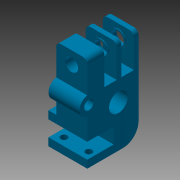
# Autodesk Inventor part: Part3
Saved by Autodesk Inventor 2015 (Build 190159000, 159)
## iProperties
Created: 2015-07-07
Part Number: Part3
Material: ABS Plastic
Document SubType Name: Modeling
Designer: eefred
Density: 1.06 g/cm^3
Appearance: Sky Blue Medium
Author: eefred
Autodesk Inventor part; units mm, degrees
ref_plane "YZ Plane" through (0, 0, 0) normal (1, 0, 0) x (0, 1, 0)
ref_plane "XZ Plane" through (0, 0, 0) normal (0, 1, 0) x (-1, 0, 0)
ref_plane "XY Plane" through (0, 0, 0) normal (0, 0, 1) x (1, 0, 0)
sketch "Sketch1" plane through (0, 0, 0) normal (1, 0, 0) x (0, 1, 0)
  line L0 (0, 0) -> (0, -5)
  line L1 (0, -5) -> (17, -5)
  line L2 (17, -5) -> (17, -15)
  line L3 (17, -15) -> (0, -15)
  line L4 (0, -61) -> (33, -61)
  line L5 (33, -61) -> (33, 0)
  line L6 (33, 0) -> (0, 0)
  circle A0 centre (1, -35) radius 3
  arc A1 (0, -29.0839) -> (0, -40.9161) centre (1, -35) ccw
  line L7 (0, -15) -> (0, -29.0839)
  line L8 (0, -61) -> (0, -40.9161)
  dimension "d0" = 5
  dimension "d1" = 17
  dimension "d2" = 10
  dimension "d4" = 33
  dimension "d6" = 6
  dimension "d7" = 1
  dimension "d8" = 20
  dimension "d9" = 6
  dimension "d49" = 46
  constraints: 18 end point, 5 perpendicular, 3 vertical, 2 centre point, 2 point on circle, 2 point on line, 1 coincident, 1 horizontal
  measures "d0" distance of L0.start L0.end
  measures "d1" distance of L0.end L1.end
  measures "d2" distance of L1.end L2.end
  measures "d4" distance of L4.start L4.end
  measures "d6" diameter of A0
  measures "d7" horizontal distance of L0.start A0.centre
  measures "d8" distance from line of L3 A0.centre
  measures "d9" radius of A1
  measures "d49" distance between parallel lines of L4 L3
extrude "Extrusion1" add sketch "Sketch1" along normal blind 25
sketch "Sketch2" plane through (0, 0, 0) normal (-1, 0, 0) x (0, 0, 1)
  line L0 (-70, -8) -> (-20, -8)
  line L1 (-20, -8) -> (-20, 42)
  line L2 (-20, 42) -> (-70, 42)
  line L3 (-70, 42) -> (-70, -8)
  point P0 (0, 0)
  dimension "d12" = 20
  dimension "d13" = 8
  dimension "d14" = 50
  dimension "d15" = 50
  constraints: 8 end point, 2 parallel, 1 horizontal, 1 perpendicular
  measures "d12" distance from line of point (0, 0) L1
  measures "d13" distance from line of point (0, 0) L0
  measures "d14" distance of L0.start L0.end
  measures "d15" distance of L2.end L0.start
extrude "Extrusion2" cut sketch "Sketch2" against normal blind 5
sketch "Sketch3" plane through (5, 0, 0) normal (-1, 0, 0) x (0, 0, 1)
  line L0 (-61, 22) -> (-40, 22)
  line L1 (-40, 22) -> (-40, 30)
  line L2 (-40, 30) -> (-61, 30)
  line L3 (-61, 30) -> (-61, 22)
  line L4 (-61, 11) -> (-40, 11)
  line L5 (-40, 11) -> (-40, 19)
  line L6 (-40, 19) -> (-61, 19)
  line L7 (-61, 19) -> (-61, 11)
  line L8 (-61, 33) -> (-20, 33) projected
  point P0 (0, 0)
  dimension "d18" = 8
  dimension "d19" = 8
  dimension "d20" = 21
  dimension "d21" = 3
  dimension "d22" = 3
  constraints: 16 end point, 4 parallel, 2 horizontal, 2 perpendicular, 2 point on line, 1 vertical alignment
  measures "d18" distance of L6.end L4.start
  measures "d19" distance of L2.end L0.start
  measures "d20" distance of L1.end L2.end
  measures "d21" distance between parallel lines of L0 L6
  measures "d22" distance between parallel lines of L8 L2
extrude "Extrusion3" cut sketch "Sketch3" against normal up to next
sketch "Sketch4" plane through (0, 33, 0) normal (0, 1, 0) x (1, 0, 0)
  circle A0 centre (15, 53) radius 4.1
  line L0 (5, 61) -> (25, 61) projected
  point P0 (0, 0)
  point P1 (15, 61)
  dimension "d25" = 8.2
  dimension "d26" = 8
  constraints: 1 centre point, 1 midpoint, 1 vertical alignment
  measures "d25" diameter of A0
  measures "d26" distance from line of L0 A0.centre
extrude "Extrusion4" cut sketch "Sketch4" against normal through all
sketch "Sketch5" plane through (5, 11, -40) normal (0, 1, 0) x (1, 0, 0)
  circle A0 centre (10, 13) radius 4.1 projected
  circle A1 centre (10, 13) radius 5
  point P0 (-5, -40)
  dimension "d29" = 10
  constraints: 1 centre point, 1 coincident
  measures "d29" diameter of A1
extrude "Extrusion5" add sketch "Sketch5" along normal blind 0.5
pattern_linear "Rectangular Pattern1" count 2 spacing 11 along (0, 1, 0) of "Extrusion5"
pattern_linear "Rectangular Pattern2" count 2 spacing 7.5 along (0, 1, 0) of "Extrusion5", "Rectangular Pattern1"
sketch "Sketch6" plane through (25, 0, 0) normal (1, 0, 0) x (0, 0, -1)
  circle A0 centre (27, 20) radius 6
  line L0 (61, 33) -> (0, 33) projected
  line L1 (0, 33) -> (0, 0) projected
  dimension "d38" = 12
  dimension "d39" = 13
  dimension "d40" = 27
  constraints: 1 centre point
  measures "d38" diameter of A0
  measures "d39" distance from line of L0 A0.centre
  measures "d40" distance from line of L1 A0.centre
extrude "Extrusion6" cut sketch "Sketch6" against normal up to surface (20 mm away)
fillet "Fillet1" radius 3 6 edges at (25, 31.5, -61) (25, 20.5, -61) (25, 5.5, -61) (5, 31.5, -61) (5, 20.5, -61) (5, 5.5, -61)
fillet "Fillet2" radius 10 1 edges at (12.5, 33, 0)
mirror "Mirror1" about plane through (0, 0, 0) normal (0, 0, 1) remove original yes
sketch "Sketch8" plane through (0, 33, 20) normal (0, 1, 0) x (1, 0, 0)
  line L0 (9.0185, 0.8332) -> (8.8914, 0.7605)
  spline S0 degree 2 poles (8.8914, 0.7605) (8.6371, 0.5971) (8.51, 0.5971) knots 0 0 0 1 1 1
  spline S1 degree 2 poles (8.51, 0.5971) (8.2557, 0.5971) (7.8925, 1.1056) (7.8925, 1.3144) knots 0 0 0 1 2 2 2
  spline S2 degree 2 poles (7.8925, 1.3144) (7.8925, 1.4052) (7.9016, 1.5505) knots 0 0 0 1 1 1
  spline S3 degree 2 poles (7.9016, 1.5505) (7.9288, 1.6958) (7.9288, 1.7321) knots 0 0 0 1 1 1
  spline S4 degree 2 poles (7.9288, 1.7321) (7.6837, 3.2668) (7.6837, 3.8842) knots 0 0 0 1 1 1
  spline S5 degree 2 poles (7.6837, 3.8842) (7.6837, 5.0465) (8.7824, 6.3996) (9.5906, 6.3996) knots 0 0 0 1 2 2 2
  spline S6 degree 2 poles (9.5906, 6.3996) (10.3624, 6.3996) (11.7518, 5.0738) (12.1967, 3.9569) knots 0 0 0 1 2 2 2
  spline S7 degree 2 poles (12.1967, 3.9569) (13.695, 5.8093) (14.258, 6.7719) knots 0 0 0 1 1 1
  spline S8 degree 2 poles (14.258, 6.7719) (14.4578, 7.1078) (14.7756, 7.1078) knots 0 0 0 1 1 1
  spline S9 degree 2 poles (14.7756, 7.1078) (14.9845, 7.1078) (15.4022, 6.6357) (15.4022, 6.4268) knots 0 0 0 1 2 2 2
  spline S10 degree 2 poles (15.4022, 6.4268) (15.4022, 6.1181) (14.8846, 5.3553) (13.7586, 3.9478) (13.6496, 3.8388) knots 0 0 0 1 2 3 3 3
  spline S11 degree 2 poles (13.6496, 3.8388) (12.8233, 2.849) (12.5509, 2.4041) knots 0 0 0 1 1 1
  spline S12 degree 2 poles (12.5509, 2.4041) (12.5509, 1.8593) (12.006, 1.8593) knots 0 0 0 1 1 1
  spline S13 degree 2 poles (12.006, 1.8593) (11.7518, 1.8593) (11.3795, 2.3405) (11.3795, 2.6584) knots 0 0 0 1 2 2 2
  spline S14 degree 2 poles (11.3795, 2.6584) (11.3795, 2.7492) (11.4067, 2.849) knots 0 0 0 1 1 1
  spline S15 degree 2 poles (11.4067, 2.849) (11.434, 2.9489) (11.434, 2.9943) knots 0 0 0 1 1 1
  spline S16 degree 2 poles (11.434, 2.9943) (11.434, 3.3212) (10.3261, 5.1283) (9.5906, 5.1283) knots 0 0 0 1 2 2 2
  spline S17 degree 2 poles (9.5906, 5.1283) (9.2274, 5.1283) (8.7098, 4.3746) (8.7098, 3.7843) knots 0 0 0 1 2 2 2
  spline S18 degree 2 poles (8.7098, 3.7843) (8.7098, 3.0942) (8.8732, 2.2497) (8.9459, 2.168) (9.2001, 2.059) (11.0798, 1.7049) (13.3318, 1.4143) (13.8585, 1.4143) knots 0 0 0 1 2 3 4 5 6 6 6
  spline S19 degree 2 poles (13.8585, 1.4143) (14.2035, 1.4143) (14.4669, 1.4688) knots 0 0 0 1 1 1
  spline S20 degree 2 poles (14.4669, 1.4688) (14.7393, 1.5142) (14.9391, 1.5142) knots 0 0 0 1 1 1
  spline S21 degree 2 poles (14.9391, 1.5142) (15.1298, 1.5142) (15.5565, 1.0693) (15.5565, 0.815) knots 0 0 0 1 2 2 2
  spline S22 degree 2 poles (15.5565, 0.815) (15.5565, 0.0885) (14.5577, 0.0885) knots 0 0 0 1 1 1
  spline S23 degree 2 poles (14.5577, 0.0885) (13.7495, 0.0885) (10.8165, 0.4518) (9.7086, 0.6969) knots 0 0 0 1 2 2 2
  spline S24 degree 2 poles (9.7086, 0.6969) (9.527, 0.7333) (9.3908, 0.7514) knots 0 0 0 1 1 1
  line L1 (9.3908, 0.7514) -> (9.0185, 0.8332)
  point P0 (0, 20)
  point P1 (7.6837, -0.6197)
  constraints: 1 other
extrude "Extrusion8" add sketch "Sketch8" along normal blind 0.5
sketch "Sketch9" plane through (0, 0, 0) normal (0, 0, -1) x (-1, 0, 0)
  circle A0 centre (-21, 5) radius 2.1
  circle A1 centre (-5, 5) radius 2.1
  line L0 (0, 0) -> (-25, 0) projected
  line L1 (0, 23) -> (0, 0) projected
  line L2 (-25, 23) -> (-25, 0) projected
  dimension "d50" = 4.2
  dimension "d51" = 5
  dimension "d52" = 5
  dimension "d53" = 4
  constraints: 2 centre point, 1 equal radius, 1 horizontal alignment
  measures "d50" diameter of A0
  measures "d51" distance from line of L0 A0.centre
  measures "d52" distance from line of L1 A1.centre
  measures "d53" distance from line of A0.centre L2
extrude "Extrusion9" cut sketch "Sketch9" against normal up to next
equation "\"d18\" = d19"
equation "\"d21\" = d22"
body "Solid1"
